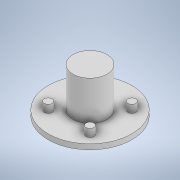
# Autodesk Inventor part: brazo_2_contra
Saved by Autodesk Inventor 2021 (Build 250183000, 183)
## iProperties
Created: 2021-10-13
Part Number: brazo_2_contra
Material: Genérico
Document SubType Name: Modeling
Designer: orgyn
Density: 1 g/cm^3
Appearance: Valor por defecto
Author: orgyn
Autodesk Inventor part; units mm, degrees
ref_plane "YZ Plane" through (0, 0, 0) normal (1, 0, 0) x (0, 1, 0)
ref_plane "XZ Plane" through (0, 0, 0) normal (0, 1, 0) x (-1, 0, 0)
ref_plane "XY Plane" through (0, 0, 0) normal (0, 0, 1) x (1, 0, 0)
sketch "Boceto1" plane through (0, 0, 0) normal (0, 1, 0) x (-1, 0, 0)
  line L0 (0, 0) -> (0, 16)
  line L1 (0, 16) -> (16, 16)
  line L2 (16, 16) -> (16, 0)
  line L3 (16, 0) -> (0, 0)
  line L4 (0, 16) -> (16, 0)
  circle A0 centre (8, 8) radius 11.3137
  circle A1 centre (16, 16) radius 1.5
  circle A2 centre (0, 16) radius 1.5
  circle A3 centre (0, 0) radius 1.5
  circle A4 centre (16, 0) radius 1.5
  circle A5 centre (8.1827, 7.8173) radius 16
  dimension "d0" = 16
  dimension "d1" = 16
  dimension "d2" = 3
  dimension "d5" = 360
  dimension "d7" = 32
  constraints: 10 end point, 5 centre point, 3 perpendicular, 1 coincident, 1 midpoint, 1 point on line, 1 vertical, 12 other
  measures "d0" distance of L0.start L0.end
  measures "d1" distance of L0.end L1.end
  measures "d2" diameter of A1
  measures "d7" diameter of A5
extrude "Extrusión1" add sketch "Boceto1" along normal blind 2 contours A3 A0 A2 L0 | L0 A2 L4 A4 L3 A3 | L3 A4 A0 A3 | A2 L1 A1 L2 A4 L4 | A0 A1 L1 A2 | L2 A1 A0 A4 | A5
sketch "Boceto2" plane through (-8.1827, 2, 7.8173) normal (0, 1, 0) x (1, 0, 0)
  point P0 (8.1827, 7.8173)
sketch "Boceto3" plane through (-8.1827, 2, 7.8173) normal (0, 1, 0) x (1, 0, 0)
  circle A0 centre (0, 0) radius 6.5
  point P0 (8.1827, 7.8173)
  dimension "d10" = 13
  constraints: 1 centre point
  measures "d10" diameter of A0
extrude "Extrusión2" add sketch "Boceto3" along normal blind 15
sketch "Boceto4" plane through (-8.1827, 0, 7.8173) normal (0, -1, 0) x (1, 0, 0)
  circle A0 centre (8.1827, 8.1827) radius 1.5 projected
  circle A1 centre (8.1827, 8.1827) radius 1.5
  circle A2 centre (8.1827, -7.8173) radius 1.5 projected
  circle A3 centre (8.1827, -7.8173) radius 1.5
  circle A4 centre (-7.8173, -7.8173) radius 1.5 projected
  circle A5 centre (-7.8173, -7.8173) radius 1.5
  circle A6 centre (-7.8173, 8.1827) radius 1.5 projected
  circle A7 centre (-7.8173, 8.1827) radius 1.5
  point P0 (8.1827, -7.8173)
  constraints: 4 centre point, 4 coincident
extrude "Extrusión3" add sketch "Boceto4" against normal blind 5
